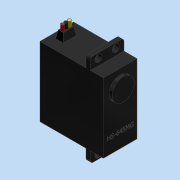
# Autodesk Inventor part: HitecServoBody
Saved by Autodesk Inventor 2017 (Build 210142000, 142)
## iProperties
Created: 2014-01-17
Part Number: HitecServoBody
Material: ABS Plastic
Document SubType Name: Modeling
Designer: Derek
Density: 1.06 g/cm^3
Appearance: Smooth - Black
Mass: 32.1533 g
Surface Area: 67.5983 cm^2
Volume: 30.3333 cm^3
Author: Derek
Autodesk Inventor part; units mm, degrees
ref_plane "YZ Plane" through (0, 0, 0) normal (1, 0, 0) x (0, 1, 0)
ref_plane "XZ Plane" through (0, 0, 0) normal (0, 1, 0) x (-1, 0, 0)
ref_plane "XY Plane" through (0, 0, 0) normal (0, 0, 1) x (1, 0, 0)
sketch "Sketch1" plane through (0, 0, 0) normal (0, 0, 1) x (1, 0, 0)
  line L0 (0, 0) -> (0, -40.64)
  line L1 (0, -40.64) -> (26.924, -40.64)
  line L2 (0, 0) -> (26.924, 0)
  line L3 (26.924, -40.64) -> (26.924, -47.244)
  line L4 (26.924, -47.244) -> (29.464, -47.244)
  line L5 (29.464, -47.244) -> (29.464, -40.64)
  line L6 (26.924, 0) -> (26.924, 6.604)
  line L7 (26.924, 6.604) -> (29.464, 6.604)
  line L8 (29.464, 6.604) -> (29.464, 0)
  line L9 (29.464, 0) -> (37.084, 0)
  line L10 (29.464, -40.64) -> (37.084, -40.64)
  line L11 (37.084, 0) -> (37.084, -40.64)
  dimension "d0" = 40.64
  dimension "d4" = 6.604
  dimension "d45" = 2.54
  dimension "d46" = 26.924
  dimension "d47" = 7.62
  dimension "d60" = 53.848
  constraints: 24 end point, 6 perpendicular, 5 equal length, 3 parallel, 2 horizontal, 1 coincident, 1 point on line, 1 vertical
  measures "d0" distance of L0.start L0.end
  measures "d4" distance of L2.end L6.end
  measures "d45" distance of L6.end L7.end
  measures "d46" distance of L0.start L2.end
  measures "d47" distance of L8.end L9.end
  measures "d60" distance between parallel lines of L4 L7
extrude "Extrusion8" add sketch "Sketch1" along normal blind 19.6342
sketch "Sketch8" plane through (37.084, -40.64, 0) normal (1, 0, 0) x (0, 0, -1)
  line L0 (0, 0) -> (0, 40.64) projected
  line L1 (0, 40.64) -> (-19.6342, 40.64) projected
  line L2 (-19.6342, 0) -> (-19.6342, 40.64) projected
  line L3 (0, 0) -> (-19.6342, 0) projected
  circle A0 centre (-9.8171, 30.861) radius 6.477
  dimension "d50" = 12.954
  dimension "d51" = 9.779
  constraints: 1 centre point
  measures "d50" diameter of A0
  measures "d51" distance from line of L1 A0.centre
extrude "Extrusion9" add sketch "Sketch8" along normal blind 1.778 contours A0
sketch "Sketch9" plane through (29.464, 0, 0) normal (1, 0, 0) x (0, 0, -1)
  circle A0 centre (-14.8971, 3.81) radius 2.1082
  line L0 (0, 6.604) -> (-19.6342, 6.604) projected
  line L1 (-9.8171, 6.604) -> (-9.8171, 8.0872)
  line L2 (0, 0) -> (-19.6342, 0) projected
  circle A1 centre (-4.7371, 3.81) radius 2.1082
  line L3 (0, 0) -> (0, -40.64) projected
  line L4 (0, -20.32) -> (8.7495, -20.32)
  circle A2 centre (-14.8971, -44.45) radius 2.1082
  circle A3 centre (-4.7371, -44.45) radius 2.1082
  dimension "d54" = 4.2164
  dimension "d55" = 5.08
  dimension "d56" = 3.81
  constraints: 4 centre point, 4 end point, 3 symmetric about line, 2 midpoint, 1 horizontal, 1 vertical, 3 other
  measures "d54" diameter of A0
  measures "d55" distance from line of L1 A0.centre
  measures "d56" distance from line of A0.centre L2
extrude "Extrusion10" cut sketch "Sketch9" against normal through all
fillet "Fillet1" radius 1.524 4 edges at (28.194, 6.604, 19.6342) (28.194, 6.604, 0) (28.194, -47.244, 19.6342) (28.194, -47.244, 0)
sketch "Sketch10" plane through (37.084, -40.64, 0) normal (1, 0, 0) x (0, 0, -1)
  line L0 (-17.5506, 9.9133) -> (-7.4594, 9.9133) construction
  line L1 (-7.4594, 9.9133) -> (-7.4594, 4.705) construction
  line L2 (-7.4594, 4.705) -> (-17.5506, 4.705) construction
  line L3 (-17.5506, 4.705) -> (-17.5506, 9.9133) construction
  line L4 (-15.5306, 7.4264) -> (-15.855, 7.4264)
  line L5 (-15.855, 7.4264) -> (-15.855, 8.6214)
  line L6 (-15.855, 8.6214) -> (-16.9788, 8.6214)
  line L7 (-16.9788, 8.6214) -> (-16.9788, 7.4264)
  line L8 (-16.9788, 7.4264) -> (-17.3033, 7.4264)
  line L9 (-17.3033, 7.4264) -> (-17.3033, 9.8678)
  line L10 (-17.3033, 9.8678) -> (-16.9788, 9.8678)
  line L11 (-16.9788, 9.8678) -> (-16.9788, 8.9103)
  line L12 (-16.9788, 8.9103) -> (-15.855, 8.9103)
  line L13 (-15.855, 8.9103) -> (-15.855, 9.8678)
  line L14 (-15.855, 9.8678) -> (-15.5306, 9.8678)
  line L15 (-15.5306, 9.8678) -> (-15.5306, 7.4264)
  spline S0 degree 2 poles (-14.3553, 7.3829) (-14.6205, 7.3829) (-14.9924, 7.4937) (-15.1566, 7.5728) knots 0 0 0 1 2 2 2
  line L16 (-15.1566, 7.5728) -> (-15.1566, 7.9804)
  line L17 (-15.1566, 7.9804) -> (-15.1329, 7.9804)
  spline S1 degree 2 poles (-15.1329, 7.9804) (-14.9726, 7.83) (-14.567, 7.6638) (-14.3791, 7.6638) knots 0 0 0 1 2 2 2
  spline S2 degree 2 poles (-14.3791, 7.6638) (-14.11, 7.6638) (-13.835, 7.8874) (-13.835, 8.0714) knots 0 0 0 1 2 2 2
  spline S3 degree 2 poles (-13.835, 8.0714) (-13.835, 8.2178) (-13.9794, 8.3998) (-14.1357, 8.4453) knots 0 0 0 1 2 2 2
  spline S4 degree 2 poles (-14.1357, 8.4453) (-14.2485, 8.477) (-14.4365, 8.5205) (-14.5769, 8.5561) knots 0 0 0 1 2 2 2
  spline S5 degree 2 poles (-14.5769, 8.5561) (-14.7036, 8.5897) (-14.9034, 8.6906) (-14.9806, 8.7718) knots 0 0 0 1 2 2 2
  spline S6 degree 2 poles (-14.9806, 8.7718) (-15.0557, 8.8529) (-15.1388, 9.0705) (-15.1388, 9.213) knots 0 0 0 1 2 2 2
  spline S7 degree 2 poles (-15.1388, 9.213) (-15.1388, 9.5097) (-14.6759, 9.9114) (-14.3178, 9.9114) knots 0 0 0 1 2 2 2
  spline S8 degree 2 poles (-14.3178, 9.9114) (-14.112, 9.9114) (-13.748, 9.8302) (-13.5917, 9.7531) knots 0 0 0 1 2 2 2
  line L18 (-13.5917, 9.7531) -> (-13.5917, 9.3653)
  line L19 (-13.5917, 9.3653) -> (-13.6154, 9.3653)
  spline S9 degree 2 poles (-13.6154, 9.3653) (-13.7321, 9.4721) (-14.0962, 9.6304) (-14.296, 9.6304) knots 0 0 0 1 2 2 2
  spline S10 degree 2 poles (-14.296, 9.6304) (-14.5215, 9.6304) (-14.8005, 9.4187) (-14.8005, 9.2466) knots 0 0 0 1 2 2 2
  spline S11 degree 2 poles (-14.8005, 9.2466) (-14.8005, 9.0923) (-14.6363, 8.9083) (-14.482, 8.8667) knots 0 0 0 1 2 2 2
  spline S12 degree 2 poles (-14.482, 8.8667) (-14.3791, 8.839) (-14.0803, 8.7678) (-13.9814, 8.7381) knots 0 0 0 1 2 2 2
  spline S13 degree 2 poles (-13.9814, 8.7381) (-13.7301, 8.661) (-13.4967, 8.3503) (-13.4967, 8.1228) knots 0 0 0 1 2 2 2
  spline S14 degree 2 poles (-13.4967, 8.1228) (-13.4967, 7.9784) (-13.6134, 7.7014) (-13.7183, 7.6045) knots 0 0 0 1 2 2 2
  spline S15 degree 2 poles (-13.7183, 7.6045) (-13.835, 7.4976) (-14.1318, 7.3829) (-14.3553, 7.3829) knots 0 0 0 1 2 2 2
  line L20 (-12.3413, 8.3464) -> (-13.2652, 8.3464)
  line L21 (-13.2652, 8.3464) -> (-13.2652, 8.6432)
  line L22 (-13.2652, 8.6432) -> (-12.3413, 8.6432)
  line L23 (-12.3413, 8.6432) -> (-12.3413, 8.3464)
  spline S16 degree 2 poles (-10.4736, 8.2178) (-10.4736, 8.0298) (-10.5982, 7.7113) (-10.7031, 7.6045) knots 0 0 0 1 2 2 2
  spline S17 degree 2 poles (-10.7031, 7.6045) (-10.8119, 7.4917) (-11.0849, 7.375) (-11.2491, 7.375) knots 0 0 0 1 2 2 2
  spline S18 degree 2 poles (-11.2491, 7.375) (-11.4133, 7.375) (-11.6844, 7.4857) (-11.7873, 7.5965) knots 0 0 0 1 2 2 2
  spline S19 degree 2 poles (-11.7873, 7.5965) (-11.9139, 7.7291) (-12.0564, 8.1743) (-12.0564, 8.4987) knots 0 0 0 1 2 2 2
  spline S20 degree 2 poles (-12.0564, 8.4987) (-12.0564, 8.8173) (-11.9258, 9.3297) (-11.7893, 9.5196) knots 0 0 0 1 2 2 2
  spline S21 degree 2 poles (-11.7893, 9.5196) (-11.6567, 9.7056) (-11.2373, 9.9133) (-10.9623, 9.9133) knots 0 0 0 1 2 2 2
  spline S22 degree 2 poles (-10.9623, 9.9133) (-10.8811, 9.9133) (-10.7387, 9.8975) (-10.6853, 9.8797) knots 0 0 0 1 2 2 2
  line L24 (-10.6853, 9.8797) -> (-10.6853, 9.5651)
  line L25 (-10.6853, 9.5651) -> (-10.6991, 9.5651)
  spline S23 degree 2 poles (-10.6991, 9.5651) (-10.7446, 9.5889) (-10.9108, 9.6304) (-11.0058, 9.6304) knots 0 0 0 1 2 2 2
  spline S24 degree 2 poles (-11.0058, 9.6304) (-11.3105, 9.6304) (-11.6844, 9.2189) (-11.72, 8.8153) knots 0 0 0 1 2 2 2
  spline S25 degree 2 poles (-11.72, 8.8153) (-11.6033, 8.8964) (-11.3579, 8.9854) (-11.2115, 8.9854) knots 0 0 0 1 2 2 2
  spline S26 degree 2 poles (-11.2115, 8.9854) (-11.0691, 8.9854) (-10.8554, 8.9281) (-10.7387, 8.841) knots 0 0 0 1 2 2 2
  spline S27 degree 2 poles (-10.7387, 8.841) (-10.6041, 8.7401) (-10.4736, 8.4275) (-10.4736, 8.2178) knots 0 0 0 1 2 2 2
  spline S28 degree 2 poles (-10.806, 8.2039) (-10.806, 8.3543) (-10.8851, 8.5581) (-10.9721, 8.6293) knots 0 0 0 1 2 2 2
  spline S29 degree 2 poles (-10.9721, 8.6293) (-11.0374, 8.6808) (-11.1997, 8.7144) (-11.2847, 8.7144) knots 0 0 0 1 2 2 2
  spline S30 degree 2 poles (-11.2847, 8.7144) (-11.3995, 8.7144) (-11.6152, 8.6451) (-11.72, 8.5798) knots 0 0 0 1 2 2 2
  spline S31 degree 2 poles (-11.72, 8.5798) (-11.722, 8.5442) (-11.7259, 8.477) (-11.7259, 8.4255) knots 0 0 0 1 2 2 2
  spline S32 degree 2 poles (-11.7259, 8.4255) (-11.7259, 8.1723) (-11.627, 7.8617) (-11.5518, 7.7805) knots 0 0 0 1 2 2 2
  spline S33 degree 2 poles (-11.5518, 7.7805) (-11.4826, 7.7034) (-11.3322, 7.642) (-11.2472, 7.642) knots 0 0 0 1 2 2 2
  spline S34 degree 2 poles (-11.2472, 7.642) (-11.0493, 7.642) (-10.806, 7.923) (-10.806, 8.2039) knots 0 0 0 1 2 2 2
  line L26 (-8.6138, 8.2653) -> (-8.9046, 8.2653)
  line L27 (-8.9046, 8.2653) -> (-8.9046, 7.4264)
  line L28 (-8.9046, 7.4264) -> (-9.2192, 7.4264)
  line L29 (-9.2192, 7.4264) -> (-9.2192, 8.2653)
  line L30 (-9.2192, 8.2653) -> (-10.2975, 8.2653)
  line L31 (-10.2975, 8.2653) -> (-10.2975, 8.6095)
  line L32 (-10.2975, 8.6095) -> (-9.2054, 9.8678)
  line L33 (-9.2054, 9.8678) -> (-8.9046, 9.8678)
  line L34 (-8.9046, 9.8678) -> (-8.9046, 8.5284)
  line L35 (-8.9046, 8.5284) -> (-8.6138, 8.5284)
  line L36 (-8.6138, 8.5284) -> (-8.6138, 8.2653)
  line L37 (-9.2192, 8.5284) -> (-9.2192, 9.482)
  line L38 (-9.2192, 9.482) -> (-10.0403, 8.5284)
  line L39 (-10.0403, 8.5284) -> (-9.2192, 8.5284)
  spline S35 degree 2 poles (-6.8727, 8.202) (-6.8727, 8.0259) (-6.9855, 7.7251) (-7.0884, 7.6143) knots 0 0 0 1 2 2 2
  spline S36 degree 2 poles (-7.0884, 7.6143) (-7.1913, 7.5036) (-7.4979, 7.375) (-7.6879, 7.375) knots 0 0 0 1 2 2 2
  spline S37 degree 2 poles (-7.6879, 7.375) (-7.862, 7.375) (-8.2023, 7.4521) (-8.3269, 7.5134) knots 0 0 0 1 2 2 2
  line L40 (-8.3269, 7.5134) -> (-8.3269, 7.8597)
  line L41 (-8.3269, 7.8597) -> (-8.3032, 7.8597)
  spline S38 degree 2 poles (-8.3032, 7.8597) (-8.2656, 7.832) (-8.1251, 7.7608) (-8.04, 7.7291) knots 0 0 0 1 2 2 2
  spline S39 degree 2 poles (-8.04, 7.7291) (-7.9431, 7.6955) (-7.7828, 7.6579) (-7.6819, 7.6579) knots 0 0 0 1 2 2 2
  spline S40 degree 2 poles (-7.6819, 7.6579) (-7.583, 7.6579) (-7.397, 7.7291) (-7.3298, 7.8063) knots 0 0 0 1 2 2 2
  spline S41 degree 2 poles (-7.3298, 7.8063) (-7.2684, 7.8795) (-7.2051, 8.0734) (-7.2051, 8.2039) knots 0 0 0 1 2 2 2
  spline S42 degree 2 poles (-7.2051, 8.2039) (-7.2051, 8.3345) (-7.2763, 8.5007) (-7.3436, 8.5561) knots 0 0 0 1 2 2 2
  spline S43 degree 2 poles (-7.3436, 8.5561) (-7.4129, 8.6174) (-7.6186, 8.6689) (-7.7433, 8.6689) knots 0 0 0 1 2 2 2
  spline S44 degree 2 poles (-7.7433, 8.6689) (-7.8778, 8.6689) (-8.1449, 8.6273) (-8.226, 8.6095) knots 0 0 0 1 2 2 2
  line L42 (-8.226, 8.6095) -> (-8.226, 9.8678)
  line L43 (-8.226, 9.8678) -> (-6.8866, 9.8678)
  line L44 (-6.8866, 9.8678) -> (-6.8866, 9.581)
  line L45 (-6.8866, 9.581) -> (-7.9114, 9.581)
  line L46 (-7.9114, 9.581) -> (-7.9114, 8.93)
  spline S45 degree 2 poles (-7.9114, 8.93) (-7.8521, 8.938) (-7.7373, 8.9439) (-7.6898, 8.9439) knots 0 0 0 1 2 2 2
  spline S46 degree 2 poles (-7.6898, 8.9439) (-7.5019, 8.9439) (-7.2427, 8.8826) (-7.124, 8.7915) knots 0 0 0 1 2 2 2
  spline S47 degree 2 poles (-7.124, 8.7915) (-7.0033, 8.7005) (-6.8727, 8.4235) (-6.8727, 8.202) knots 0 0 0 1 2 2 2
  line L47 (-4.3581, 7.4264) -> (-4.6825, 7.4264)
  line L48 (-4.6825, 7.4264) -> (-4.6825, 9.5295)
  line L49 (-4.6825, 9.5295) -> (-5.3196, 8.0991)
  line L50 (-5.3196, 8.0991) -> (-5.5175, 8.0991)
  line L51 (-5.5175, 8.0991) -> (-6.1486, 9.5295)
  line L52 (-6.1486, 9.5295) -> (-6.1486, 7.4264)
  line L53 (-6.1486, 7.4264) -> (-6.4513, 7.4264)
  line L54 (-6.4513, 7.4264) -> (-6.4513, 9.8678)
  line L55 (-6.4513, 9.8678) -> (-6.0081, 9.8678)
  line L56 (-6.0081, 9.8678) -> (-5.3988, 8.5086)
  line L57 (-5.3988, 8.5086) -> (-4.8092, 9.8678)
  line L58 (-4.8092, 9.8678) -> (-4.3581, 9.8678)
  line L59 (-4.3581, 9.8678) -> (-4.3581, 7.4264)
  spline S48 degree 2 poles (-2.8406, 7.3789) (-3.0998, 7.3789) (-3.5291, 7.5372) (-3.6834, 7.6974) knots 0 0 0 1 2 2 2
  spline S49 degree 2 poles (-3.6834, 7.6974) (-3.8377, 7.8597) (-4.0019, 8.3385) (-4.0019, 8.6491) knots 0 0 0 1 2 2 2
  spline S50 degree 2 poles (-4.0019, 8.6491) (-4.0019, 8.9439) (-3.8358, 9.4108) (-3.6814, 9.577) knots 0 0 0 1 2 2 2
  spline S51 degree 2 poles (-3.6814, 9.577) (-3.533, 9.7373) (-3.0978, 9.9114) (-2.8386, 9.9114) knots 0 0 0 1 2 2 2
  spline S52 degree 2 poles (-2.8386, 9.9114) (-2.714, 9.9114) (-2.4884, 9.8758) (-2.3855, 9.8441) knots 0 0 0 1 2 2 2
  spline S53 degree 2 poles (-2.3855, 9.8441) (-2.3024, 9.8204) (-2.1006, 9.7333) (-2.0393, 9.7016) knots 0 0 0 1 2 2 2
  line L60 (-2.0393, 9.7016) -> (-2.0393, 9.3099)
  line L61 (-2.0393, 9.3099) -> (-2.067, 9.3099)
  spline S54 degree 2 poles (-2.067, 9.3099) (-2.1283, 9.3633) (-2.2569, 9.4603) (-2.3756, 9.5157) knots 0 0 0 1 2 2 2
  spline S55 degree 2 poles (-2.3756, 9.5157) (-2.4746, 9.5651) (-2.7298, 9.6304) (-2.8762, 9.6304) knots 0 0 0 1 2 2 2
  spline S56 degree 2 poles (-2.8762, 9.6304) (-3.2284, 9.6304) (-3.6636, 9.1002) (-3.6636, 8.659) knots 0 0 0 1 2 2 2
  spline S57 degree 2 poles (-3.6636, 8.659) (-3.6636, 8.4137) (-3.5489, 8.0457) (-3.4401, 7.919) knots 0 0 0 1 2 2 2
  spline S58 degree 2 poles (-3.4401, 7.919) (-3.3352, 7.7924) (-3.0384, 7.6599) (-2.8524, 7.6599) knots 0 0 0 1 2 2 2
  spline S59 degree 2 poles (-2.8524, 7.6599) (-2.7159, 7.6599) (-2.4429, 7.6994) (-2.3499, 7.739) knots 0 0 0 1 2 2 2
  line L62 (-2.3499, 7.739) -> (-2.3499, 8.3701)
  line L63 (-2.3499, 8.3701) -> (-2.9158, 8.3701)
  line L64 (-2.9158, 8.3701) -> (-2.9158, 8.655)
  line L65 (-2.9158, 8.655) -> (-2.0294, 8.655)
  line L66 (-2.0294, 8.655) -> (-2.0294, 7.5886)
  spline S60 degree 2 poles (-2.0294, 7.5886) (-2.0907, 7.5609) (-2.3005, 7.4759) (-2.3895, 7.4501) knots 0 0 0 1 2 2 2
  spline S61 degree 2 poles (-2.3895, 7.4501) (-2.5102, 7.4145) (-2.7041, 7.3789) (-2.8406, 7.3789) knots 0 0 0 1 2 2 2
  point P0 (0, 40.64)
  dimension "d0" = 40.64
  dimension "d4" = 6.604
  dimension "d45" = 2.54
  dimension "d46" = 26.924
  dimension "d47" = 7.62
  dimension "d60" = 53.848
  constraints: 2 other
emboss "Emboss1" sketch "Sketch10" operation cut depth 0.254 direction (-1, 0, 0)
sketch "Sketch11" plane through (0, 0, 0) normal (0, 1, 0) x (1, 0, 0)
  line L0 (7.62, -6.0071) -> (3.175, -6.0071)
  line L1 (3.175, -6.0071) -> (3.175, -13.6271)
  line L2 (3.175, -13.6271) -> (7.62, -13.6271)
  line L3 (7.62, -13.6271) -> (7.62, -6.0071)
  line L4 (0, 0) -> (0, -19.6342) projected
  point P0 (7.62, -9.8171)
  point P1 (0, -9.8171)
  dimension "d63" = 7.62
  dimension "d64" = 4.445
  dimension "d65" = 3.175
  constraints: 8 end point, 2 midpoint, 2 parallel, 1 horizontal, 1 horizontal alignment, 1 perpendicular
  measures "d63" distance of L2.end L0.start
  measures "d64" distance of L0.start L0.end
  measures "d65" distance between parallel lines of L4 L1
extrude "Extrusion11" add sketch "Sketch11" along normal blind 4.445
chamfer "Chamfer2" distance 0.762 distance2 4.445 1 edges at (5.3975, 4.445, 6.0071) measured on face at (4.6567, 4.445, 8.5471)
chamfer "Chamfer3" distance 0.762 distance2 4.445 1 edges at (3.175, 4.445, 10.1981) measured on face at (4.6567, 4.445, 9.055)
chamfer "Chamfer4" distance 0.762 distance2 4.445 1 edges at (5.7785, 4.445, 13.6271) measured on face at (5.1646, 4.445, 9.055)
chamfer "Chamfer5" distance 0.762 distance2 4.445 1 edges at (7.62, 4.445, 9.8171) measured on face at (5.1646, 4.445, 8.8011)
sketch "Sketch12" plane through (0, 4.445, 0) normal (0, 1, 0) x (1, 0, 0)
  line L0 (6.858, -6.7691) -> (6.858, -12.8651) projected
  line L1 (3.937, -6.7691) -> (6.858, -6.7691) projected
  line L2 (3.937, -12.8651) -> (3.937, -6.7691) projected
  line L3 (6.858, -12.8651) -> (3.937, -12.8651) projected
  circle A0 centre (5.3975, -9.8171) radius 0.9525
  circle A1 centre (5.3975, -11.8227) radius 0.9525
  circle A2 centre (5.3975, -7.849) radius 0.9525
  line L4 (6.858, -12.8651) -> (3.937, -12.8651) projected
  point P0 (0, 0)
  point P1 (3.937, -9.8171)
  point P2 (5.3975, -12.8651)
  point P3 (5.3975, -12.8651)
  point P4 (5.3975, -12.8651)
  dimension "d80" = 1.905
  constraints: 4 midpoint, 3 centre point, 3 vertical alignment, 2 equal radius, 1 horizontal alignment
  measures "d80" diameter of A0
extrude "Extrusion12" add sketch "Sketch12" along normal blind 3.175 contours A0 | A1 | A2
body "Solid2"
